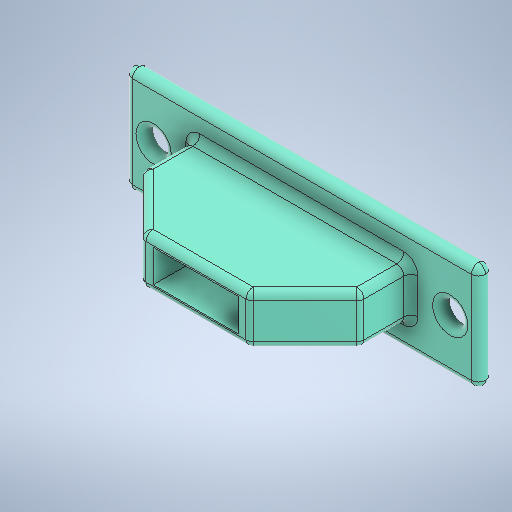
# Autodesk Inventor part: Usb_DOCK_ControlHub_DplyHub
Saved by Autodesk Inventor 2025.1 (Build 291241000, 241)
## iProperties
Created: 2024-08-19
Part Number: Usb_DOCK_ControlHub_DplyHub
Material: Generic
Document SubType Name: Modeling
Designer: shubh
Density: 1 g/cm^3
Appearance: Default
Author: shubh
Autodesk Inventor part; units mm, degrees
ref_plane "YZ Plane" through (0, 0, 0) normal (1, 0, 0) x (0, 1, 0)
ref_plane "XZ Plane" through (0, 0, 0) normal (0, 1, 0) x (-1, 0, 0)
ref_plane "XY Plane" through (0, 0, 0) normal (0, 0, 1) x (1, 0, 0)
sketch "Sketch1" plane through (0, 0, 0) normal (0, 0, 1) x (1, 0, 0)
  line L0 (-25, 7.5) -> (25, 7.5)
  line L1 (25, 7.5) -> (25, -7.5)
  line L2 (25, -7.5) -> (-25, -7.5)
  line L3 (-25, -7.5) -> (-25, 7.5)
  line L4 (-25, 7.5) -> (25, -7.5) construction
  line L5 (25, 7.5) -> (-25, -7.5) construction
  line L6 (0, 7.5) -> (0, -7.5) construction
  line L7 (-25, 0) -> (25, 0) construction
  circle A0 centre (-21, 0) radius 1.5
  circle A1 centre (21, 0) radius 1.5
  point P0 (0, 0)
  dimension "d0" = 50
  dimension "d1" = 15
  dimension "d2" = 3
  dimension "d3" = 45
  constraints: 16 end point, 6 midpoint, 2 centre point, 2 parallel, 1 horizontal, 1 perpendicular, 1 point on line, 1 symmetric about line, 1 other
  measures "d0" distance of L1.end L2.end
  measures "d1" distance of L0.end L1.end
  measures "d2" diameter of A0
extrude "Extrusion1" add sketch "Sketch1" along normal blind 2
sketch "Sketch2" plane through (0, 0, 2) normal (0, 0, 1) x (1, 0, 0)
  line L0 (-25, -7.5) -> (25, -7.5) projected
  line L1 (25, -7.5) -> (25, 7.5) projected
  line L2 (25, 7.5) -> (-25, 7.5) projected
  line L3 (-25, 7.5) -> (-25, -7.5) projected
  circle A0 centre (21, 0) radius 1.5 projected
  circle A1 centre (-21, 0) radius 1.5 projected
  line L4 (0, 7.5) -> (0, -7.5) construction
  line L5 (-25, 0) -> (25, 0) construction
  line L6 (7.5, -3.5) -> (-7.5, -3.5)
  line L7 (-7.5, -3.5) -> (-7.5, 3.5)
  line L8 (-7.5, 3.5) -> (7.5, 3.5)
  line L9 (7.5, 3.5) -> (7.5, -3.5)
  line L10 (7.5, -3.5) -> (-7.5, 3.5) construction
  line L11 (-7.5, -3.5) -> (7.5, 3.5) construction
  line L12 (-7.5, 3.5) -> (-15.4306, 3.5)
  line L13 (-15.4306, 3.5) -> (-15.4306, -3.5)
  line L14 (-15.4306, -3.5) -> (-7.5, -3.5)
  line L15 (-7.5, -3.5) -> (-7.5, 3.5)
  line L16 (7.5, -3.5) -> (7.5, 3.5)
  line L17 (-7.5, 3.5) -> (-7.5, -3.5)
  line L18 (7.5, 3.5) -> (15.4306, 3.5)
  line L19 (15.4306, 3.5) -> (15.4306, -3.5)
  line L20 (15.4306, -3.5) -> (7.5, -3.5)
  line L21 (7.5, -3.5) -> (7.5, 3.5)
  line L22 (7.5, 3.5) -> (15.4306, 3.5)
  line L23 (15.4306, 3.5) -> (15.4306, -3.5)
  line L24 (15.4306, -3.5) -> (7.5, -3.5)
  point P0 (0, 0)
  point P1 (7.5, -3.5)
  dimension "d6" = 15
  dimension "d7" = 7
  constraints: 42 end point, 10 symmetric about line, 6 midpoint, 4 parallel, 2 horizontal, 2 perpendicular
  measures "d6" distance of L7.end L8.end
  measures "d7" distance of L8.end L6.start
extrude "Extrusion2" add sketch "Sketch2" along normal blind 15 contours L6 L7 L8 L9 | L9 L18 L19 L20 | L14 L13 L12 L7
sketch "Sketch3" plane through (0, 0, 17) normal (0, 0, 1) x (1, 0, 0)
  line L0 (-15.4306, -3.5) -> (-15.4306, 3.5) projected
  line L1 (-15.4306, 3.5) -> (15.4306, 3.5) projected
  line L2 (15.4306, 3.5) -> (15.4306, -3.5) projected
  line L3 (15.4306, -3.5) -> (-15.4306, -3.5) projected
  line L4 (-25, -7.5) -> (25, -7.5) projected
  line L5 (25, -7.5) -> (25, 7.5) projected
  line L6 (25, 7.5) -> (-25, 7.5) projected
  line L7 (-25, 7.5) -> (-25, -7.5) projected
  circle A0 centre (21, 0) radius 1.5 projected
  circle A1 centre (-21, 0) radius 1.5 projected
  line L8 (-15.4306, -3.5) -> (15.4306, -3.5) projected
  line L9 (15.4306, -3.5) -> (15.4306, 3.5) projected
  line L10 (15.4306, 3.5) -> (-15.4306, 3.5) projected
  line L11 (-15.4306, 3.5) -> (-15.4306, -3.5) projected
  line L12 (0, 3.5) -> (0, -3.5) construction
  line L13 (-15.4306, 0) -> (15.4306, 0) construction
  line L14 (6.05, -2.3) -> (-6.05, -2.3)
  line L15 (-6.05, -2.3) -> (-6.05, 2.3)
  line L16 (-6.05, 2.3) -> (6.05, 2.3)
  line L17 (6.05, 2.3) -> (6.05, -2.3)
  line L18 (6.05, -2.3) -> (-6.05, 2.3) construction
  line L19 (-6.05, -2.3) -> (6.05, 2.3) construction
  point P0 (0, 0)
  dimension "d10" = 12.1
  dimension "d11" = 4.6
  constraints: 16 end point, 6 midpoint, 2 parallel, 1 horizontal, 1 perpendicular
  measures "d10" distance of L15.end L16.end
  measures "d11" distance of L14.end L15.end
extrude "Extrusion3" cut sketch "Sketch3" against normal blind 11.5 contours L14 L15 L16 L17
chamfer "Chamfer1" distance 7.9375 angle 45 2 edges at (15.4306, 0, 17) (-15.4306, 0, 17)
fillet "Fillet1" radius 1 34 edges at (-15.4306, 0, 2) (15.4306, 0, 9.0625) (11.4619, 3.5, 13.0312) (11.4619, -3.5, 13.0312) (15.4306, 0, 2) (15.4306, -3.5, 5.5312) (15.4306, 3.5, 5.5312) (0, -3.5, 2) (0, 3.5, 2) (0, 7.5, 2) (0, -7.5, 2) (0, 7.5, 0) (0, -7.5, 0) (19.5, 0, 2) (19.5, 0, 0) (25, -7.5, 1) (25, 0, 2) (-15.4306, -3.5, 5.5312) (-15.4306, 3.5, 5.5312) (-7.4931, 0, 17) (-11.4619, 3.5, 13.0312) (-11.4619, -3.5, 13.0312) (-15.4306, 0, 9.0625) (-22.5, 0, 0) (-22.5, 0, 2) (7.4931, 0, 17) (0, 3.5, 17) (0, -3.5, 17) (25, 7.5, 1) (-25, 0, 2) (-25, -7.5, 1) (-25, 7.5, 1) (-25, 0, 0) (25, 0, 0)
body "Solid1"
